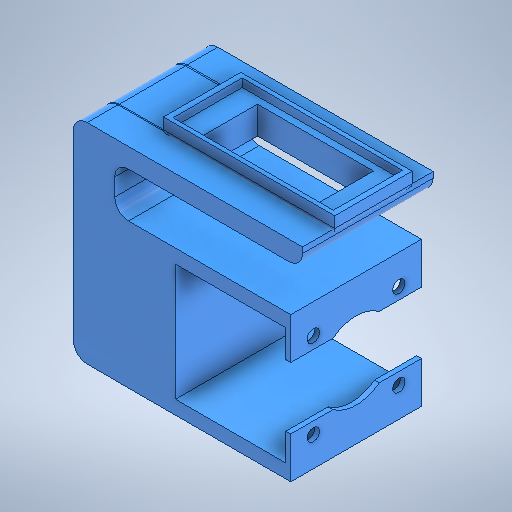
# Autodesk Inventor part: Attache moteur côté rocker
Saved by Autodesk Inventor 2026.2 (Build 302298010, 298A)
## iProperties
Created: 2026-03-22
Part Number: Attache moteur côté rocker
Material: Générique
Document SubType Name: Modeling
Designer: Genon
Density: 1 g/cm^3
Appearance: Cyan
Author: Genon
Autodesk Inventor part; units mm, degrees
ref_plane "XY Plane" through (0, 0, 0) normal (0, 0, 1) x (1, 0, 0)
sketch "Esquisse1" plane through (0, 0, 0) normal (0, 1, 0) x (-1, 0, 0)
  line L0 (-21, 10.05) -> (21, 10.05)
  line L1 (21, 10.05) -> (21, -10.05)
  line L2 (21, -10.05) -> (-21, -10.05)
  line L3 (-21, -10.05) -> (-21, 10.05)
  line L4 (-21, 10.05) -> (21, -10.05) construction
  line L5 (21, 10.05) -> (-21, -10.05) construction
  line L6 (-29, 12.5) -> (29, 12.5)
  line L7 (29, 12.5) -> (29, -12.5)
  line L8 (29, -12.5) -> (-29, -12.5)
  line L9 (-29, -12.5) -> (-29, 12.5)
  line L10 (-29, 12.5) -> (29, -12.5) construction
  line L11 (29, 12.5) -> (-29, -12.5) construction
  point P0 (0, 0)
  dimension "d0" = 42
  dimension "d1" = 20.1
  dimension "d2" = 58
  dimension "d3" = 25
  constraints: 24 end point, 4 midpoint, 4 parallel, 2 horizontal, 2 perpendicular
  measures "d0" distance of L1.end L2.end
  measures "d1" distance of L0.end L1.end
  measures "d2" distance of L7.end L8.end
  measures "d3" distance of L6.end L7.end
extrude "Extrusion1" add sketch "Esquisse1" along normal blind 10
sketch "Esquisse3" plane through (0, 10, 0) normal (0, 1, 0) x (1, 0, 0)
  line L0 (29, 12.5) -> (-29, 12.5) projected
  line L1 (-29, 12.5) -> (-29, -12.5) projected
  line L2 (-29, -12.5) -> (29, -12.5) projected
  line L3 (29, -12.5) -> (29, 12.5) projected
  line L4 (-31, -14) -> (31, -14)
  line L5 (31, -14) -> (31, 14)
  line L6 (31, 14) -> (-31, 14)
  line L7 (-31, 14) -> (-31, -14)
  line L8 (-31, -14) -> (31, 14) construction
  line L9 (31, -14) -> (-31, 14) construction
  point P0 (0, 0)
  dimension "d12" = 62
  dimension "d13" = 28
  constraints: 12 end point, 2 midpoint, 2 parallel, 1 horizontal, 1 perpendicular
  measures "d12" distance of L6.end L5.end
  measures "d13" distance of L5.end L4.end
extrude "Extrusion3" add sketch "Esquisse3" along normal mid plane 6
fillet "Congé1" radius 2 4 edges at (0, 7, 14) (-31, 7, 0) (0, 7, -14) (31, 7, 0)
sketch "Esquisse4" plane through (-29, 0, -12.5) normal (-1, 0, 0) x (0, 0, 1)
  line L0 (24.5, 7) -> (0.5, 7) projected
  arc A0 (0, 7.0635) -> (0.5, 7) centre (0.5, 9) ccw projected
  line L1 (0, 7.0635) -> (0, 0) projected
  line L2 (0, 0) -> (25, 0) projected
  line L3 (25, 0) -> (25, 7.0635) projected
  arc A1 (24.5, 7) -> (25, 7.0635) centre (24.5, 9) ccw projected
  point P0 (12.5, 0)
extrude "Extrusion4" add sketch "Esquisse4" along normal blind 25
sketch "Esquisse5" plane through (0, 0, 0) normal (0, -1, 0) x (1, 0, 0)
  line L0 (29, 12.5) -> (-54, 12.5) projected
  line L1 (29, -12.5) -> (-54, -12.5) projected
  line L2 (-54, 12.5) -> (-39, 12.5)
  line L3 (-39, 12.5) -> (-39, -12.5)
  line L4 (-39, -12.5) -> (-54, -12.5)
  line L5 (-54, -12.5) -> (-54, 12.5)
  point P0 (0, 0)
  dimension "d19" = 15
  constraints: 8 end point, 2 parallel, 1 horizontal, 1 perpendicular, 1 point on line
  measures "d19" distance of L3.end L4.end
extrude "Extrusion5" add sketch "Esquisse5" along normal blind 42.5
fillet "Congé2" radius 5 4 edges at (-39, 0, 0) (-54, 7.0159, -12.252) (-54, 7.0159, 12.252) (-54, 7, 0)
fillet "Congé3" radius 5 1 edges at (29, 0, 0)
sketch "Esquisse6" plane through (0, -42.5, 0) normal (0, -1, 0) x (1, 0, 0)
  line L0 (-54, -12.5) -> (-39, -12.5) projected
  line L1 (-39, -12.5) -> (-39, 12.5) projected
  line L2 (-39, 12.5) -> (-54, 12.5) projected
  line L3 (-54, 12.5) -> (-54, -12.5) projected
  point P0 (0, 0)
extrude "Extrusion6" add sketch "Esquisse6" along normal blind 21.15
ref_plane "Plan de construction1" through (0, -42.5, 0) normal (0, 1, 0) x (-1, 0, 0)
sketch "Esquisse7" plane through (0, -63.65, 0) normal (0, -1, 0) x (1, 0, 0)
  line L0 (-39, -12.5) -> (-39, 12.5) projected
  line L1 (-39, 12.5) -> (-54, 12.5) projected
  line L2 (-54, 12.5) -> (-54, -12.5) projected
  line L3 (-54, -12.5) -> (-39, -12.5) projected
  point P0 (0, 0)
extrude "Extrusion7" add sketch "Esquisse7" along normal blind 5
ref_plane "Plan de construction2" through (-39, 0, 0) normal (1, 0, 0) x (0, 1, 0)
fillet "Congé4" radius 5 1 edges at (-54, -68.65, 0)
ref_plane "Plan de construction3" through (0, -21.3, 0) normal (0, 1, 0) x (-1, 0, 0)
ref_plane "Plan de construction4" through (0, -63.7, 0) normal (0, 1, 0) x (-1, 0, 0)
sketch "Esquisse10" plane through (0, -63.7, 0) normal (0, 1, 0) x (-1, 0, 0)
  line L0 (39, -12.5) -> (39, 12.5) projected
  line L1 (39, -12.5) -> (-23, -12.5)
  line L2 (-23, -12.5) -> (-23, 12.5)
  line L3 (-23, 12.5) -> (39, 12.5)
  line L4 (39, 12.5) -> (39, -12.5)
  point P0 (0, 0)
  dimension "d38" = 62
  constraints: 8 end point, 2 parallel, 1 horizontal, 1 perpendicular
  measures "d38" distance of L2.end L3.end
extrude "Extrusion10" add sketch "Esquisse10" against normal blind 5
sketch "Esquisse11" plane through (0, -63.7, 0) normal (0, 1, 0) x (-1, 0, 0)
  line L0 (39, -12.5) -> (-23, -12.5) projected
  line L1 (-23, -12.5) -> (-24.75, -12.5)
  line L2 (-24.75, -12.5) -> (-24.75, 12.5)
  line L3 (-24.75, 12.5) -> (-23, 12.5)
  line L4 (-23, 12.5) -> (-23, -12.5)
  point P0 (0, 0)
  dimension "d41" = 1.75
  dimension "d42" = 25
  constraints: 8 end point, 2 parallel, 1 horizontal, 1 perpendicular
  measures "d41" distance of L2.end L3.end
  measures "d42" distance of L1.end L2.end
sketch "Esquisse12" plane through (23, -63.7, 12.5) normal (1, 0, 0) x (0, 0, -1)
  line L0 (0, 0) -> (25, 0) projected
  line L1 (0, 0) -> (0, -5) projected
  line L2 (25, -5) -> (0, -5) projected
  line L3 (25, 0) -> (25, -5) projected
  point P0 (12.5, 63.7)
extrude "Extrusion11" add sketch "Esquisse12" along normal blind 1.75
extrude "Extrusion12" add sketch "Esquisse11" along normal blind 10
sketch "Esquisse13" plane through (0, -21.3, 0) normal (0, 1, 0) x (-1, 0, 0)
  line L0 (-23, 12.5) -> (-23, -12.5) projected
  line L1 (-23, -12.5) -> (39, -12.5) projected
  line L2 (39, 12.5) -> (39, -12.5) projected
  line L3 (39, 12.5) -> (-23, 12.5) projected
  point P0 (0, 0)
extrude "Extrusion13" add sketch "Esquisse13" along normal blind 5
fillet "Congé5" radius 5 1 edges at (-39, -16.3, 0)
sketch "Esquisse14" plane through (23, -21.3, 12.5) normal (1, 0, 0) x (0, 0, -1)
  line L0 (0, 0) -> (25, 0) projected
  line L1 (25, 0) -> (25, 5) projected
  line L2 (0, 5) -> (25, 5) projected
  line L3 (0, 0) -> (0, 5) projected
  point P0 (12.5, 21.3)
extrude "Extrusion14" add sketch "Esquisse14" along normal blind 1.75
sketch "Esquisse15" plane through (0, -21.3, 0) normal (0, -1, 0) x (1, 0, 0)
  line L0 (-34, 12.5) -> (24.75, 12.5) projected
  line L1 (-34, -12.5) -> (24.75, -12.5) projected
  line L2 (24.75, 12.5) -> (23, 12.5)
  line L3 (23, 12.5) -> (23, -12.5)
  line L4 (23, -12.5) -> (24.75, -12.5)
  line L5 (24.75, -12.5) -> (24.75, 12.5)
  point P0 (0, 0)
  point P1 (24.75, -12.5)
  dimension "d52" = 1.75
  constraints: 8 end point, 2 parallel, 1 horizontal, 1 perpendicular, 1 point on line
  measures "d52" distance of L4.end L3.end
extrude "Extrusion15" add sketch "Esquisse15" along normal blind 10
ref_plane "Plan de construction5" through (9, 0, 0) normal (1, 0, 0) x (0, 1, 0)
sketch "Esquisse17" plane through (-29.5, 7.0635, 12.5) normal (0, 0, 1) x (1, 0, 0)
  arc A0 (-24.5, -70.7135) -> (-19.5, -75.7135) centre (-19.5, -70.7135) ccw projected
  line L0 (-9.5, -75.7135) -> (-19.5, -75.7135) projected
  line L1 (-9.5, -75.7135) -> (-9.5, -75.7635) projected
  line L2 (-9.5, -75.7635) -> (54.25, -75.7635) projected
  line L3 (54.25, -75.7635) -> (54.25, -60.7635) projected
  line L4 (52.5, -60.7635) -> (54.25, -60.7635) projected
  line L5 (52.5, -70.7635) -> (52.5, -60.7635) projected
  line L6 (-9.5, -70.7635) -> (52.5, -70.7635) projected
  line L7 (-9.5, -28.3635) -> (-9.5, -70.7635) projected
  line L8 (-9.5, -28.3635) -> (52.5, -28.3635) projected
  line L9 (52.5, -28.3635) -> (52.5, -38.3635) projected
  line L10 (54.25, -38.3635) -> (52.5, -38.3635) projected
  line L11 (54.25, -23.3635) -> (54.25, -38.3635) projected
  line L12 (-4.5, -23.3635) -> (54.25, -23.3635) projected
  arc A1 (-9.5, -18.3635) -> (-4.5, -23.3635) centre (-4.5, -18.3635) ccw projected
  line L13 (-9.5, -12.0635) -> (-9.5, -18.3635) projected
  arc A2 (-4.5, -7.0635) -> (-9.5, -12.0635) centre (-4.5, -12.0635) ccw projected
  line L14 (53.5, -7.0635) -> (-4.5, -7.0635) projected
  arc A3 (53.5, -7.0635) -> (58.5, -2.0635) centre (53.5, -2.0635) ccw projected
  line L15 (58.5, -2.0635) -> (58.5, 0) projected
  line L16 (0, 0) -> (58.5, 0) projected
  line L17 (0, 0) -> (-19.5, 0) projected
  spline S0 degree 6 poles (-24.5, -5.0456) (-24.5, -4.7068) (-24.4726, -4.3679) (-24.4178, -4.0318) (-24.336, -3.7013) (-24.228, -3.3789) (-23.9561, -2.7418) (-23.7898, -2.428) (-23.5974, -2.1288) (-23.3807, -1.8467) (-23.1417, -1.5842) (-22.7649, -1.2341) (-22.6432, -1.1293) (-22.5175, -1.0292) (-22.3881, -0.9339) (-22.2553, -0.8436) (-22.0724, -0.7292) (-22.0252, -0.7005) (-21.9776, -0.6724) (-21.9297, -0.645) (-21.8814, -0.6182) (-21.7691, -0.5578) (-21.7049, -0.5247) (-21.64, -0.4927) (-21.5747, -0.4618) (-21.5088, -0.432) (-21.352, -0.3644) (-21.2607, -0.3276) (-21.1685, -0.2929) (-21.0756, -0.2604) (-20.9818, -0.2302) (-20.6627, -0.1355) (-20.4341, -0.0816) (-20.2026, -0.0409) (-19.9691, -0.0136) (-19.7345, 0) (-19.5, 0) knots 0 0 0 0 0 0 0 0.257896 0.257896 0.257896 0.257896 0.257896 0.52724 0.52724 0.52724 0.52724 0.52724 0.649449 0.649449 0.649449 0.649449 0.649449 0.691501 0.691501 0.691501 0.691501 0.691501 0.746535 0.746535 0.746535 0.746535 0.746535 0.821498 0.821498 0.821498 0.821498 0.821498 1 1 1 1 1 1 1 projected
  line L18 (-24.5, -5.0456) -> (-24.5, -70.7135) projected
  point P0 (29.5, -7.0635)
  constraints: 1 other
extrude "Extrusion16" add sketch "Esquisse17" along normal blind 11.15
sketch "Esquisse18" plane through (29, 7.0635, -12.5) normal (0, 0, -1) x (-1, 0, 0)
  arc A0 (78, -75.7135) -> (83, -70.7135) centre (78, -70.7135) ccw projected
  line L0 (83, -5.0456) -> (83, -70.7135) projected
  spline S0 degree 6 poles (78, 0) (78.2345, 0) (78.4691, -0.0136) (78.7026, -0.0409) (78.9341, -0.0816) (79.1627, -0.1355) (79.4818, -0.2302) (79.5756, -0.2604) (79.6685, -0.2929) (79.7607, -0.3276) (79.852, -0.3644) (80.0088, -0.432) (80.0747, -0.4618) (80.14, -0.4927) (80.2049, -0.5247) (80.2691, -0.5578) (80.3814, -0.6182) (80.4297, -0.645) (80.4776, -0.6724) (80.5252, -0.7005) (80.5724, -0.7292) (80.7553, -0.8436) (80.8881, -0.9339) (81.0175, -1.0292) (81.1432, -1.1293) (81.2649, -1.2341) (81.6417, -1.5842) (81.8807, -1.8467) (82.0974, -2.1288) (82.2898, -2.428) (82.4561, -2.7418) (82.728, -3.3789) (82.836, -3.7013) (82.9178, -4.0318) (82.9726, -4.3679) (83, -4.7068) (83, -5.0456) knots 0 0 0 0 0 0 0 0.178502 0.178502 0.178502 0.178502 0.178502 0.253465 0.253465 0.253465 0.253465 0.253465 0.308499 0.308499 0.308499 0.308499 0.308499 0.350551 0.350551 0.350551 0.350551 0.350551 0.47276 0.47276 0.47276 0.47276 0.47276 0.742104 0.742104 0.742104 0.742104 0.742104 1 1 1 1 1 1 1 projected
  line L1 (58.5, 0) -> (78, 0) projected
  line L2 (58.5, 0) -> (0, 0) projected
  line L3 (0, 0) -> (0, -2.0635) projected
  arc A1 (0, -2.0635) -> (5, -7.0635) centre (5, -2.0635) ccw projected
  line L4 (5, -7.0635) -> (63, -7.0635) projected
  arc A2 (68, -12.0635) -> (63, -7.0635) centre (63, -12.0635) ccw projected
  line L5 (68, -12.0635) -> (68, -18.3635) projected
  arc A3 (63, -23.3635) -> (68, -18.3635) centre (63, -18.3635) ccw projected
  line L6 (63, -23.3635) -> (4.25, -23.3635) projected
  line L7 (4.25, -23.3635) -> (4.25, -38.3635) projected
  line L8 (6, -38.3635) -> (4.25, -38.3635) projected
  line L9 (6, -28.3635) -> (6, -38.3635) projected
  line L10 (68, -28.3635) -> (6, -28.3635) projected
  line L11 (68, -28.3635) -> (68, -70.7635) projected
  line L12 (6, -70.7635) -> (68, -70.7635) projected
  line L13 (6, -70.7635) -> (6, -60.7635) projected
  line L14 (4.25, -60.7635) -> (6, -60.7635) projected
  line L15 (4.25, -75.7635) -> (4.25, -60.7635) projected
  line L16 (68, -75.7635) -> (4.25, -75.7635) projected
  line L17 (68, -75.7135) -> (68, -75.7635) projected
  line L18 (78, -75.7135) -> (68, -75.7135) projected
  point P0 (29, -7.0635)
  constraints: 1 other
extrude "Extrusion17" add sketch "Esquisse18" along normal blind 11.15
sketch "Esquisse19" plane through (9, 0, 0) normal (1, 0, 0) x (0, 1, 0)
  line L0 (-21.3, -23.65) -> (-21.3, 23.65) projected
  line L1 (-63.7, 23.65) -> (-21.3, 23.65) projected
  line L2 (-63.7, 23.65) -> (-63.7, -23.65) projected
  line L3 (-21.3, -23.65) -> (-63.7, -23.65) projected
  line L4 (-21.3, 23.65) -> (-42.5, 23.65)
  line L5 (-42.5, 23.65) -> (-42.5, -23.65)
  line L6 (-42.5, 0) -> (-27, 0)
  line L7 (-27, 0) -> (-27, -15.5)
  line L8 (-27, -15.5) -> (-58, -15.5)
  line L9 (-58, -15.5) -> (-58, 15.5)
  line L10 (-58, 15.5) -> (-27, 15.5)
  point P0 (0, 0)
  dimension "d63" = 15.5
  dimension "d64" = 15.5
  dimension "d65" = 31
  dimension "d66" = 31
  constraints: 14 end point, 4 coincident, 4 perpendicular, 3 midpoint, 1 horizontal, 1 point on line
  measures "d63" distance of L6.start L6.end
  measures "d64" distance of L6.end L7.end
  measures "d65" distance of L7.end L8.end
  measures "d66" distance of L8.end L9.end
hole "Perçage1" at (9, -27, 15.5) at (9, -27, -15.5) at (9, -58, -15.5) at (9, -58, 15.5) direction (1, 0, 0) diameter 4.5 end through all
sketch "Esquisse20" plane through (24.75, -21.3, 12.5) normal (1, 0, 0) x (0, 0, -1)
  line L0 (36.15, -10) -> (-11.15, -10) projected
  line L1 (-11.15, -10) -> (12.5, -10)
  line L2 (12.5, -10) -> (23.5, -10)
  line L3 (12.5, -10) -> (1.5, -10)
  line L4 (12.5, -10) -> (12.5, -32.4)
  line L5 (-11.15, -32.4) -> (36.15, -32.4) projected
  circle A0 centre (12.5, -21.2) radius 14
  circle A1 centre (12.5, -21.2) radius 11
  point P0 (12.5, 21.3)
  point P1 (4.1, -32.4)
  point P2 (20.9, -32.4)
  point P3 (20.9, -10)
  point P4 (4.1, -10)
  dimension "d76" = 28
  dimension "d77" = 22
  constraints: 8 end point, 3 midpoint, 2 centre point, 2 point on line, 1 coincident
  measures "d76" diameter of A0
  measures "d77" diameter of A1
extrude "Extrusion18" cut sketch "Esquisse20" against normal blind 5 contours L0 A0 | A0 L5
sketch "Esquisse21" plane through (-39, -63.7, 23.65) normal (1, 0, 0) x (0, 0, -1)
  line L0 (47.3, 42.4) -> (0, 42.4) projected
  line L1 (0, 0) -> (0, 42.4) projected
  line L2 (0, 0) -> (47.3, 0) projected
  line L3 (47.3, 42.4) -> (47.3, 0) projected
  point P0 (23.65, 63.7)
extrude "Extrusion19" add sketch "Esquisse21" along normal blind 22
